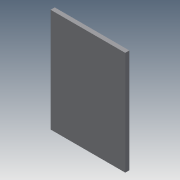
# Autodesk Inventor part: guardplate
Saved by Autodesk Inventor 2015 (Build 190159000, 159)
## iProperties
Created: 2014-08-31
Part Number: guardplate
Material: Generic
Document SubType Name: Modeling
Designer: shohei
Density: 1 g/cm^3
Appearance: Default
Author: shohei
Autodesk Inventor part; units mm, degrees
ref_plane "YZ Plane" through (0, 0, 0) normal (1, 0, 0) x (0, 1, 0)
ref_plane "XZ Plane" through (0, 0, 0) normal (0, 1, 0) x (-1, 0, 0)
ref_plane "XY Plane" through (0, 0, 0) normal (0, 0, 1) x (1, 0, 0)
sketch "Block1" plane through (0, 0, 0) normal (0, 0, 1) x (1, 0, 0)
  line L0 (0.22, -250.22) -> (-180.22, -250.22)
  line L1 (-180.22, -250.22) -> (-180.22, 0.22)
  line L2 (-180.22, 0.22) -> (0.22, 0.22)
  line L3 (0.22, 0.22) -> (0.22, -250.22)
  circle A0 centre (-10, -230) radius 2.72
  circle A1 centre (-10, -20) radius 2.72
  circle A2 centre (-170, -20) radius 2.72
  circle A3 centre (-170, -230) radius 2.72
  point P0 (-90, -125)
sketch "Sketch1" plane through (0, 0, 0) normal (0, 1, 0) x (-1, 0, 0)
  line L0 (0, 0) -> (180, 0)
  line L1 (180, 0) -> (180, 250)
  line L2 (180, 250) -> (0, 250)
  line L3 (0, 250) -> (0, 0)
  circle A0 centre (170, 230) radius 2.5
  line L4 (90, 267.688) -> (90, -13.7422)
  line L5 (215.5014, 125) -> (-35.5429, 125)
  circle A1 centre (10, 230) radius 2.5
  circle A2 centre (170, 20) radius 2.5
  circle A3 centre (10, 20) radius 2.5
  dimension "d1" = 250
  dimension "d2" = 180
  dimension "d5" = 5
  dimension "d6" = 10
  dimension "d7" = 20
  dimension "d8" = 90
  dimension "d9" = 125
  constraints: 12 end point, 4 centre point, 3 symmetric about line, 2 horizontal, 2 parallel, 1 perpendicular, 1 vertical, 3 other
  measures "d1" distance of L0.end L1.end
  measures "d2" distance of L1.end L2.end
  measures "d5" diameter of A0
  measures "d6" distance from line of L1 A0.centre
  measures "d7" distance from line of L2 A0.centre
  measures "d8" distance between parallel lines of L3 L4
  measures "d9" distance between parallel lines of L0 L5
extrude "Extrusion2" add sketch "Sketch1" along normal blind 10
sketch "Sketch2" plane through (0, 10, 0) normal (0, 1, 0) x (1, 0, 0)
  circle A0 centre (-10, -20) radius 2.5 projected
  circle A1 centre (-170, -20) radius 2.5 projected
  circle A2 centre (-10, -230) radius 2.5 projected
  circle A3 centre (-170, -230) radius 2.5 projected
  line L0 (0, 0) -> (-180, 0) projected
  line L1 (-180, 0) -> (-180, -250) projected
  line L2 (-180, -250) -> (0, -250) projected
  line L3 (0, -250) -> (0, 0) projected
  constraints: 3 perpendicular, 4 other
sketch "DXF" plane through (0, 0, 0) normal (0, 1, 0) x (-1, 0, 0)
  point P0 (0, 0)
body "Solid2"
